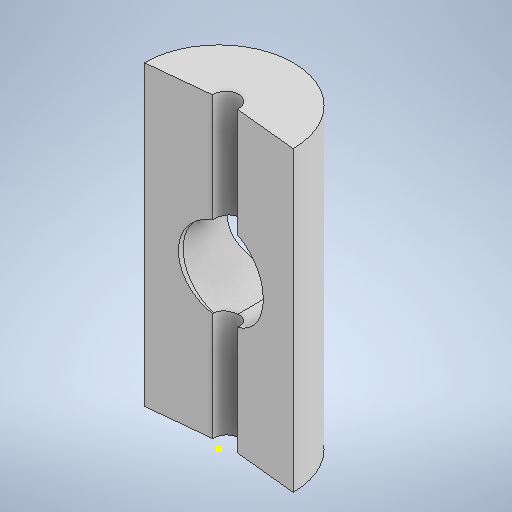
# Autodesk Inventor part: joy part1
Saved by Autodesk Inventor 2025.2 (Build 292293000, 293)
## iProperties
Created: 2025-03-25
Part Number: joy part1
Material: Generic
Document SubType Name: Modeling
Designer: avnr2
Density: 1 g/cm^3
Appearance: Default
Author: avnr2
Autodesk Inventor part; units mm, degrees
ref_plane "YZ Plane" through (0, 0, 0) normal (1, 0, 0) x (0, 1, 0)
ref_plane "XZ Plane" through (0, 0, 0) normal (0, 1, 0) x (-1, 0, 0)
ref_plane "XY Plane" through (0, 0, 0) normal (0, 0, 1) x (1, 0, 0)
sketch "Sketch1" plane through (0, 0, 0) normal (0, 1, 0) x (-1, 0, 0)
  point P0 (0, 0)
sketch "Sketch2" plane through (0, 0, 0) normal (0, 1, 0) x (-1, 0, 0)
  arc A0 (-15, 0.0122) -> (15, 0) centre (0, 0) ccw
  line L0 (15, 0) -> (2.4876, -1.2512)
  line L1 (-2.4874, -1.2492) -> (-15, 0.0122)
  arc A1 (-2.4874, -1.2492) -> (2.4876, -1.2512) centre (0, -1.5) ccw
  dimension "d0" = 1.5
  dimension "d1" = 30
  dimension "d2" = 5
  constraints: 4 end point, 4 point on circle, 2 centre point, 2 coincident, 1 vertical alignment
  measures "d0" distance of point (0, 0) point (0, -1.5)
  measures "d1" diameter of A0
  measures "d2" diameter of A1
extrude "Extrusion1" add sketch "Sketch2" along normal blind 60
sketch "Sketch3" plane through (-2.4876, 0, -1.2512) normal (0.0995, 0, 0.995) x (0.995, 0, -0.0995)
  circle A0 centre (2.3507, 30) radius 8.5
  line L0 (17.2751, 0) -> (17.2751, 60) projected
  point P0 (2.3507, 0)
  point P1 (17.2751, 30)
  dimension "d5" = 17
  constraints: 1 centre point, 1 horizontal alignment, 1 midpoint
  measures "d5" diameter of A0
extrude "Extrusion2" cut sketch "Sketch3" against normal blind 35
sketch "Sketch4" plane through (15, 0, 0.0122) normal (-0.1003, 0, 0.995) x (0.995, 0, 0.1003)
  ellipse E0 centre (-15.2223, 30) end of major axis (-15.2223, 38.5) minor radius 8.3303 (-12.6259, 21.9234) -> (-12.6259, 38.0766) ccw projected
  circle A0 centre (-15.2223, 30) radius 8.5
  point P0 (-14.9256, 0)
  constraints: 1 centre point, 1 coincident, 2 other
extrude "Extrusion3" cut sketch "Sketch4" along normal blind 35
sketch "Sketch5" plane through (2.4874, 0, -1.2492) normal (-0.1003, 0, 0.995) x (0.995, 0, 0.1003)
  ellipse E0 centre (-2.6463, 30) end of major axis (-2.6463, 38.5) minor radius 8.3303 (-0.0499, 21.9234) -> (-0.0499, 38.0766) ccw projected
  circle A0 centre (-2.6463, 30) radius 8.5
  point P0 (-2.3495, 0)
  constraints: 1 centre point, 1 coincident, 2 other
extrude "Extrusion4" cut sketch "Sketch5" against normal blind 35
sketch "Sketch6" plane through (0, 0, 0) normal (0, -1, 0) x (1, 0, 0)
  point P0 (0, 0)
body "Solid1"
